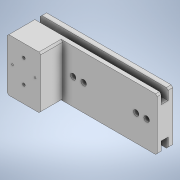
# Autodesk Inventor part: 711C-1-APP-mount
Saved by Autodesk Inventor 2020 (Build 240168000, 168)
## iProperties
ItemSpecifications: {"_id":"6046a6511c60850009bae100","finish":"543ef1f380da5b0c476373c1","finish_location":null,"material":"5515e170db035c20ce34af9a","process_initialism":null,"quotes":null,"current_quote":null,"quantity_ordered":1,"features":null,"hardware":null,"threading":{"quantity":2},"part_markings":[],"surface_roughness":null,"tolerance":null,"weld_quantity":null,"Notes":" :: Thread Spec: 2x See Notes/Drawing :: \r\n","certifications":[],"part":null,"revision_num":0,"last_history":null,"inspection_requirement_details":{"inspection_requirement":"std","customer_data_sheet":null},"feedback":null}
ItemSpecifications: {"_id":"6046a2d3e45be3000966158c","finish":"543ef1f380da5b0c476373c1","finish_location":null,"material":"5515e170db035c20ce34af9a","process_initialism":null,"quotes":null,"current_quote":null,"quantity_ordered":1,"features":null,"hardware":null,"threading":{"quantity":2},"part_markings":[],"surface_roughness":null,"tolerance":null,"weld_quantity":null,"Notes":" :: Thread Spec: 2x See Notes/Drawing :: \r\n","certifications":[],"part":null,"revision_num":0,"last_history":null,"inspection_requirement_details":{"inspection_requirement":"std","customer_data_sheet":null},"feedback":null}
Created: 2021-02-18
Part Number: 711C-1-APP-mount
Material: Generic
Document SubType Name: Modeling
Designer: maria
Density: 1 g/cm^3
Appearance: Default
Author: maria
Autodesk Inventor part; units mm, degrees
ref_plane "YZ Plane" through (0, 0, 0) normal (1, 0, 0) x (0, 1, 0)
ref_plane "XZ Plane" through (0, 0, 0) normal (0, 1, 0) x (-1, 0, 0)
ref_plane "XY Plane" through (0, 0, 0) normal (0, 0, 1) x (1, 0, 0)
sketch "Sketch1" plane through (0, 0, 0) normal (0, 0, 1) x (1, 0, 0)
  line L0 (-40.45, 31.75) -> (114.3, 31.75)
  line L1 (114.3, 31.75) -> (114.3, -31.75)
  line L2 (114.3, -31.75) -> (-40.45, -31.75)
  line L3 (-40.45, -31.75) -> (-40.45, 31.75)
  point P0 (0, 0)
  dimension "d0" = 63.5
  dimension "d1" = 31.75
  dimension "d2" = 40.45
  dimension "LENGTH" = 154.75
  constraints: 8 end point, 2 parallel, 1 horizontal, 1 perpendicular
  measures "d0" distance of L2.end L0.start
  measures "d1" vertical distance of L0.start point (0, 0)
  measures "d2" distance from line of L3 point (0, 0)
  measures "LENGTH" distance of L0.start L0.end
extrude "Extrusion1" add sketch "Sketch1" along normal blind 18.9
sketch "Sketch2" plane through (0, 0, 18.9) normal (0, 0, 1) x (1, 0, 0)
  line L0 (114.3, 31.75) -> (-40.45, 31.75) projected
  line L1 (-40.45, -31.75) -> (114.3, -31.75) projected
  line L2 (-40.45, 31.75) -> (0, 31.75)
  line L3 (0, 31.75) -> (0, -31.75)
  line L4 (0, -31.75) -> (-40.45, -31.75)
  line L5 (-40.45, -31.75) -> (-40.45, 31.75)
  point P0 (0, 0)
  dimension "d6" = 40.45
  constraints: 8 end point, 2 parallel, 1 horizontal, 1 perpendicular, 1 point on line
  measures "d6" distance between parallel lines of L5 L3
extrude "Extrusion2" add sketch "Sketch2" along normal blind 26.759
sketch "Sketch3" plane through (0, 0, 0) normal (0, 0, 1) x (1, 0, 0)
  line L0 (114.3, -31.75) -> (114.3, 31.75) projected
  point P0 (0, 0)
  point P1 (12.7, 0)
  point P2 (25.4, 0)
  point P3 (88.9, 0)
  point P4 (101.6, 0)
  dimension "d9" = 0
  dimension "d10" = 0
  dimension "d11" = 0
  dimension "d12" = 0
  dimension "d13" = 88.9
  dimension "d14" = 12.7
  dimension "d15" = 63.5
  dimension "d16" = 12.7
  measures "d9" vertical distance of point (25.4, 0) point (12.7, 0)
  measures "d10" vertical distance of point (101.6, 0) point (88.9, 0)
  measures "d11" vertical distance of point (25.4, 0) point (88.9, 0)
  measures "d12" vertical distance of point (0, 0) point (25.4, 0)
  measures "d13" distance of point (101.6, 0) point (12.7, 0)
  measures "d14" distance from line of L0 point (101.6, 0)
  measures "d15" distance of point (25.4, 0) point (88.9, 0)
  measures "d16" distance of point (101.6, 0) point (88.9, 0)
hole "Hole2" at (12.7, 0, 0) at (101.6, 0, 0) at (25.4, 0, 0) at (88.9, 0, 0) direction (0, 0, 1) diameter 6.7 end through all counterbore diameter 11 counterbore depth 6.4 clearance for "Socket Head Cap Screw" size "1/4" standard "Ansi Unified Screw Threads"
sketch "Sketch4" plane through (-40.45, -31.75, 0) normal (0, -1, 0) x (1, 0, 0)
  line L0 (0, 5.775) -> (154.75, 5.775)
  line L1 (154.75, 5.775) -> (154.75, 14.125)
  line L2 (154.75, 14.125) -> (0, 14.125)
  line L3 (0, 14.125) -> (0, 5.775)
  line L4 (0, 5.775) -> (154.75, 14.125) construction
  line L5 (154.75, 5.775) -> (0, 14.125) construction
  line L6 (0, 0) -> (0, 45.659) projected
  line L7 (0, 0) -> (154.75, 0) projected
  point P0 (40.45, 0)
  point P1 (77.375, 9.95)
  dimension "d31" = 154.75
  dimension "d32" = 77.375
  dimension "d33" = 9.95
  dimension "SLOT_HEIGHT" = 8.35
  constraints: 12 end point, 2 midpoint, 2 parallel, 1 horizontal, 1 perpendicular
  measures "d31" distance of L1.end L2.end
  measures "d32" distance from line of L6 point (77.375, 9.95)
  measures "d33" distance from line of L7 point (77.375, 9.95)
  measures "SLOT_HEIGHT" distance of L0.end L1.end
sketch "Sketch5" plane through (-40.45, 31.75, 0) normal (0, 1, 0) x (1, 0, 0)
  line L0 (154.75, -5.775) -> (0, -5.775)
  line L1 (0, -5.775) -> (0, -14.125)
  line L2 (0, -14.125) -> (154.75, -14.125)
  line L3 (154.75, -14.125) -> (154.75, -5.775)
  line L4 (154.75, -5.775) -> (0, -14.125) construction
  line L5 (0, -5.775) -> (154.75, -14.125) construction
  line L6 (0, 0) -> (0, -45.659) projected
  point P0 (40.45, 0)
  point P1 (77.375, -9.95)
  dimension "d35" = 8.35
  dimension "d36" = 154.75
  dimension "d37" = 0
  dimension "d38" = 9.95
  constraints: 12 end point, 2 midpoint, 2 parallel, 1 horizontal, 1 perpendicular
  measures "d35" distance of L2.end L0.start
  measures "d36" distance of L1.end L2.end
  measures "d37" distance between parallel lines of L6 L1
  measures "d38" vertical distance of L6.start point (77.375, -9.95)
extrude "Extrusion3" cut sketch "Sketch5" against normal blind 12.7
extrude "Extrusion4" cut sketch "Sketch4" against normal blind 12.7
sketch "Sketch6" plane through (0, 0, 45.659) normal (0, 0, 1) x (1, 0, 0)
  line L0 (0, 31.75) -> (-40.45, 31.75) projected
  line L1 (-40.45, -31.75) -> (0, -31.75) projected
  line L2 (-40.45, 31.75) -> (-40.45, -31.75) projected
  line L3 (-6.575, 2.048) -> (-6.575, 3.048) construction
  line L4 (-5.525, 2.048) -> (-5.525, 3.048)
  line L5 (-7.625, 3.048) -> (-7.625, 2.048)
  arc A0 (-7.625, 2.048) -> (-5.525, 2.048) centre (-6.575, 2.048) ccw
  arc A1 (-5.525, 3.048) -> (-7.625, 3.048) centre (-6.575, 3.048) ccw
  point P0 (0, 0)
  point P1 (-20.225, -11.502)
  point P2 (-20.225, 16.598)
  point P3 (-33.875, 2.548)
  point P4 (-6.575, 2.548)
  dimension "d43" = 0
  dimension "d44" = 15.152
  dimension "d45" = 0
  dimension "d46" = 20.248
  dimension "d47" = 20.225
  dimension "d48" = 28.1
  dimension "d50" = 27.3
  dimension "d51" = 14.05
  dimension "d52" = 13.65
  dimension "d67" = 1.05
  dimension "d68" = 1
  constraints: 8 end point, 4 point on circle, 4 tangent, 2 centre point, 1 midpoint, 1 parallel, 1 vertical
  measures "d43" vertical distance of point (-6.575, 2.548) point (-33.875, 2.548)
  measures "d44" distance from line of L0 point (-20.225, 16.598)
  measures "d45" horizontal distance of point (-20.225, -11.502) point (-20.225, 16.598)
  measures "d46" distance from line of L1 point (-20.225, -11.502)
  measures "d47" distance from line of point (-20.225, 16.598) L2
  measures "d48" distance of point (-20.225, 16.598) point (-20.225, -11.502)
  measures "d50" distance of point (-6.575, 2.548) point (-33.875, 2.548)
  measures "d51" vertical distance of point (-33.875, 2.548) point (-20.225, -11.502)
  measures "d52" horizontal distance of point (-20.225, -11.502) point (-33.875, 2.548)
  measures "d67" radius of A1
  measures "d68" distance of L3.start L3.end
hole "Hole3" at (-33.875, 2.548, 45.659) at (-6.575, 2.548, 45.659) direction (0, 0, -1) diameter 2.1 depth 4.1
hole "Hole4" at (-20.225, -11.502, 45.659) at (-20.225, 16.598, 45.659) direction (0, 0, -1) diameter 3.302 depth 12.3 thread size "8-32 UNC" class "2B" standard "ANSI Unified Screw Threads"
chamfer "Chamfer1" [suppressed]
chamfer "Chamfer2" distance 2 angle 45 10 edges at (0, -31.75, 32.2795) (-40.45, -31.75, 29.892) (-40.45, -31.75, 2.8875) (114.3, -31.75, 16.5125) (114.3, -31.75, 2.8875) (114.3, 31.75, 16.5125) (114.3, 31.75, 2.8875) (0, 31.75, 32.2795) (-40.45, 31.75, 29.892) (-40.45, 31.75, 2.8875)
equation "\"d0\" = WIDTH"
equation "\"d1\" = 0.5 * WIDTH"
equation "\"d2\" = APP_LENGTH"
equation "\"LENGTH\" = APP_LENGTH + ISOLATOR_MT_LENGTH"
equation "\"d6\" = APP_LENGTH"
equation "\"d7\" = APP_HEIGHT"
equation "\"d31\" = LENGTH"
equation "\"d32\" = 0.5 * LENGTH"
equation "\"d33\" = 0.5 * ISOLATOR_HEIGHT"
equation "\"d35\" = SLOT_HEIGHT"
equation "\"d36\" = LENGTH"
equation "\"d38\" = 0.5 * ISOLATOR_HEIGHT"
equation "\"d41\" = SLOT_DEPTH"
equation "\"d51\" = 0.5 * d48"
equation "\"d52\" = 0.5 * d50"
equation "\"ISOLATOR_MT_LENGTH\" = 114.3"
equation "\"WIDTH\" = 63.5"
equation "\"ISOLATOR_HEIGHT\" = 19.9"
equation "\"APP_LENGTH\" = 40.45"
equation "\"APP_HEIGHT\" = 26.759"
equation "\"SLOT_DEPTH\" = 12.7"
body "Solid1"
